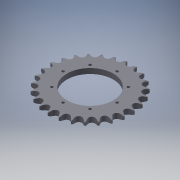
# Autodesk Inventor part: Roller Chain Sprocket1
Saved by Autodesk Inventor 2016 (Build 200138000, 138)
## iProperties
Created: 2016-05-10
Part Number: Roller Chain Sprocket1
Material: Steel
Document SubType Name: Modeling
Designer: hesaon
Density: 1 g/cm^3
Appearance: Steel
CustomPartVersion: 1
Author: hesaon
Autodesk Inventor part; units mm, degrees
ref_plane "YZ Plane" through (0, 0, 0) normal (1, 0, 0) x (0, 1, 0)
ref_plane "XZ Plane" through (0, 0, 0) normal (0, 1, 0) x (-1, 0, 0)
ref_plane "XY Plane" through (0, 0, 0) normal (0, 0, 1) x (1, 0, 0)
sketch "Theoretical Tooth Profile" plane through (0, 0, 0) normal (0, 0, 1) x (1, 0, 0)
  circle A0 centre (0, 0) radius 41.0232 construction
  line L0 (0, 0) -> (0, 41.0232) construction
  line L1 (0, 0) -> (9.4606, 39.9174) construction
  circle A1 centre (0, 0) radius 43.6033
  arc A2 (-2.5535, 39.0834) -> (2.5535, 39.0834) centre (0, 41.0232) ccw
  line L2 (0, 41.0232) -> (9.4606, 39.9174) construction
  line L3 (0, 41.0232) -> (4.0452, 44.0961) construction
  line L4 (4.0452, 44.0961) -> (-3.6757, 41.0864) construction
  arc A3 (4.846, 43.3332) -> (3.9849, 41.8797) centre (8.8299, 39.9911) ccw
  arc A4 (-3.9849, 41.8797) -> (-4.846, 43.3332) centre (-8.8299, 39.9911) ccw
  line L5 (-8.8299, 39.9911) -> (-3.9849, 41.8797) construction
  arc A5 (-3.6757, 41.0864) -> (-2.5535, 39.0834) centre (4.0452, 44.0961) ccw
  line L6 (-3.6757, 41.0864) -> (-3.9849, 41.8797)
  arc A6 (2.5535, 39.0834) -> (3.6757, 41.0864) centre (-4.0452, 44.0961) ccw
  line L7 (3.9849, 41.8797) -> (3.6757, 41.0864)
  line L8 (0, 0) -> (5.062, 43.3085) construction
  point P0 (4.7303, 40.4703)
  dimension "d0" = 82.0464
  dimension "d2" = 13.333
  dimension "d3" = 3.2067
  dimension "d10" = 127.222
  dimension "d11" = 15.926
  dimension "d12" = 5.08
  dimension "d13" = 8.2867
  dimension "d14" = 8.89
  dimension "d23" = 2.8575
  constraints: 18 end point, 15 point on circle, 7 centre point, 3 coincident, 3 point on line, 3 symmetric about line, 3 tangent, 1 equal radius, 1 midpoint, 1 parallel, 1 vertical, 1 other
  measures "d0" diameter of A0
  measures "d2" angle of L1 L0
  measures "d3" radius of A2
  measures "d10" angle of L3 L0
  measures "d11" angle of L4 L3
  measures "d12" distance of L2.start L3.end
  measures "d13" distance of L3.end L4.end
  measures "d14" distance of A3.centre L0.end
  measures "d23" distance from line of L8.end L2
sketch "Tooth Profile" plane through (0, 0, 0) normal (0, 0, 1) x (1, 0, 0)
  arc A0 (-2.9802, 39.8392) -> (2.9802, 39.8392) centre (0, 41.0232) ccw
  arc A1 (4.7477, 43.344) -> (2.9802, 39.8392) centre (23.5169, 31.6805) ccw
  arc A2 (-2.9802, 39.8392) -> (-4.7477, 43.344) centre (-23.5169, 31.6805) ccw
  line L0 (0, 0) -> (0, 41.0232) construction
  line L1 (0, 41.0232) -> (2.9802, 39.8392) construction
  line L2 (0, 41.0232) -> (-2.9802, 39.8392) construction
  circle A3 centre (0, 0) radius 43.6033 projected
  dimension "d44" = 136.667
  dimension "d45" = 22.098
  dimension "d46" = 3.2067
  constraints: 9 point on circle, 6 end point, 3 centre point, 2 tangent, 1 coincident, 1 equal radius, 1 vertical, 1 other
  measures "d44" angle of L2 L1
  measures "d45" radius of A1
  measures "d46" radius of A0
sketch "Section Profile" plane through (0, 0, 0) normal (1, 0, 0) x (0, 1, 0)
  line L0 (43.6033, 0) -> (-43.6033, 0) projected
  line L1 (32.2696, 2.6598) -> (-32.2696, 2.6598)
  line L2 (-32.2696, 2.6598) -> (-32.2696, -2.6598)
  line L3 (-32.2696, -2.6598) -> (32.2696, -2.6598)
  line L4 (32.2696, -2.6598) -> (32.2696, 2.6598)
  line L5 (32.2696, 2.6598) -> (43.6033, 2.6598) construction
  line L6 (43.6033, 2.6598) -> (43.6033, -2.6598) construction
  line L7 (43.6033, -2.6598) -> (32.2696, -2.6598) construction
  line L8 (32.2696, -2.6598) -> (32.2696, 2.6598)
  arc A0 (43.6033, 1.4692) -> (38.992, 2.6598) centre (38.992, -6.8652) ccw
  arc A1 (38.992, -2.6598) -> (43.6033, -1.4692) centre (38.992, 6.8652) ccw
  line L9 (38.992, 2.6598) -> (0, 2.6598)
  line L10 (0, 2.6598) -> (0, -2.6598)
  line L11 (0, -2.6598) -> (38.992, -2.6598)
  line L12 (0, 2.6598) -> (0, -2.6598)
  line L13 (43.6033, 1.4692) -> (43.6033, -1.4692)
  point P0 (0, 0)
  point P1 (0, 0)
  dimension "d30" = 5.3196
  dimension "d31" = 64.5392
  dimension "d32" = 5.3196
  dimension "d33" = 1.1906
  dimension "d34" = 9.525
  dimension "d43" = 2.6598
  constraints: 26 end point, 7 midpoint, 5 perpendicular, 4 parallel, 4 point on circle, 3 point on line, 3 symmetric about line, 2 centre point, 2 horizontal, 2 tangent, 1 collinear, 1 other
  measures "d30" distance between parallel lines of L7 L5
  measures "d31" distance between parallel lines of L2 L4
  measures "d32" distance between parallel lines of L3 L1
  measures "d33" distance from line of L13.start L5
  measures "d34" radius of A0
  measures "d43" distance between parallel lines of L3 L0
revolve "Shroud" add sketch "Section Profile" angle 360 about axis through (0, 0, 2.6598) along (0, 0, -1) contours L10 L3 L2 L0 | L0 L2 L1 L10
revolve "Strand" add sketch "Section Profile" angle 360 about axis through (0, 0, 2.6598) along (0, 0, -1) contours L13 A1 L11 L4 L0 | L0 L4 L9 A0 L13 | L4 L3 L10 L0 | L0 L10 L1 L4
pattern_of_one "Strand Pattern"
extrude "Theoretical Tooth" cut sketch "Theoretical Tooth Profile" along normal through all both and the other way through all contours A3 L7 A6 A2 A5 L6 A4 A1 picked at (0, 41.6543)
extrude "Tooth" [suppressed]
pattern_circular "Tooth Pattern" count 27 over 360 about axis through (0, 0, -10) along (0, 0, 1) of "Theoretical Tooth"
ref_plane "Timing Plane" through (0, 41.0232, 0) normal (1, 0, 0) x (0, 1, 0)
sketch "Sketch4" plane through (0, 41.0232, 2.6598) normal (0, 0, 1) x (1, 0, 0)
  circle A0 centre (0, -41.0232) radius 24
  circle A1 centre (0, -13.0232) radius 1.4
  circle A2 centre (-19.799, -21.2242) radius 1.4
  circle A3 centre (-28, -41.0232) radius 1.4
  circle A4 centre (-19.799, -60.8222) radius 1.4
  circle A5 centre (0, -69.0232) radius 1.4
  circle A6 centre (19.799, -60.8222) radius 1.4
  circle A7 centre (28, -41.0232) radius 1.4
  circle A8 centre (19.799, -21.2242) radius 1.4
  dimension "d51" = 48
  dimension "d52" = 2.8
  dimension "d53" = 0
  dimension "d54" = 28
  dimension "d57" = 360
  constraints: 9 centre point, 1 coincident, 17 other
  measures "d51" diameter of A0
  measures "d52" diameter of A1
  measures "d53" horizontal distance of point (0, -41.023) A1.centre
  measures "d54" distance of point (0, -41.023) A1.centre
extrude "Extrusion4" cut sketch "Sketch4" against normal through all
equation "\"d3\" = 0.5 * da_Dr + da_SC"
equation "\"d12\" = 0.8 * da_Dr"
equation "\"d13\" = 1.3 * da_Dr + da_SC"
equation "\"d14\" = 1.4 * da_Dr"
equation "\"d23\" = da_Ha"
equation "\"d44\" = da_Alfa"
equation "\"d45\" = da_Re"
equation "\"d46\" = da_Ri"
equation "\"d30\" = da_Bf"
equation "\"d31\" = da_Ds"
equation "\"d32\" = da_Bs"
equation "\"d33\" = da_Ba"
equation "\"d34\" = da_Rx"
equation "\"d40\" = da_pt"
equation "\"form_type\" = 0"
equation "\"da_p\" = 9.525"
equation "\"da_Dr\" = 6.35"
equation "\"da_SC\" = 0.03175"
equation "\"da_Ha\" = 2.8575"
equation "\"da_pt\" = 10.24"
equation "\"da_Bf\" = 5.3196"
equation "\"da_Ba\" = 1.19063"
equation "\"da_Rx\" = 9.525"
equation "\"da_Ra\" = 0.381"
equation "\"da_Bs\" = 5.3196"
equation "\"da_Ds\" = 64.53918"
equation "\"da_Re\" = 22.098"
equation "\"da_Ri\" = 3.20675"
equation "\"da_Alfa\" = 136.667deg"
body "Solid1"
